Autodesk Inventor part; units mm, degrees
(part 3 of 3)
  line L1793 (-13.4182, -23.4177) -> (-13.3812, -23.2649)
  line L1794 (-13.3812, -23.2649) -> (-13.3062, -22.9928)
  line L1795 (-13.3062, -22.9928) -> (-13.2108, -22.6965)
  line L1796 (-13.2108, -22.6965) -> (-13.192, -22.6208)
  line L1797 (-13.192, -22.6208) -> (-13.1819, -22.5545)
  line L1798 (-13.1819, -22.5545) -> (-13.1803, -22.4978)
  line L1799 (-13.1803, -22.4978) -> (-13.1866, -22.4511)
  line L1800 (-13.1866, -22.4511) -> (-13.2004, -22.4146)
  line L1801 (-13.2004, -22.4146) -> (-13.2213, -22.3887)
  line L1802 (-13.2213, -22.3887) -> (-13.2509, -22.37)
  line L1803 (-13.2509, -22.37) -> (-13.4263, -22.2651)
  line L1804 (-13.4263, -22.2651) -> (-13.601, -22.1589)
  line L1805 (-13.601, -22.1589) -> (-13.6314, -22.1414)
  line L1806 (-13.6314, -22.1414) -> (-13.664, -22.135)
  line L1807 (-13.664, -22.135) -> (-13.7027, -22.1398)
  line L1808 (-13.7027, -22.1398) -> (-13.747, -22.1561)
  line L1809 (-13.747, -22.1561) -> (-13.7963, -22.184)
  line L1810 (-13.7963, -22.184) -> (-13.8503, -22.2238)
  line L1811 (-13.8503, -22.2238) -> (-13.9085, -22.2757)
  line L1812 (-13.9085, -22.2757) -> (-14.126, -22.4984)
  line L1813 (-14.126, -22.4984) -> (-14.3317, -22.6917)
  line L1814 (-14.3317, -22.6917) -> (-14.4495, -22.7958)
  line L1815 (-14.4495, -22.7958) -> (-14.5782, -22.9048)
  line L1816 (-14.5782, -22.9048) -> (-14.7187, -23.0187)
  line L1817 (-14.7187, -23.0187) -> (-14.8697, -23.1361)
  line L1818 (-14.8697, -23.1361) -> (-15.0319, -23.2568)
  line L1819 (-15.0319, -23.2568) -> (-15.2066, -23.3812)
  line L1820 (-15.2066, -23.3812) -> (-15.393, -23.5081)
  line L1821 (-15.393, -23.5081) -> (-15.5922, -23.6378)
  line L1822 (-15.5922, -23.6378) -> (-15.7628, -23.7441)
  arc A47 (-16.4074, -23.3034) -> (-15.7628, -23.7441) centre (0, 0) ccw
  line L1823 (-16.4074, -23.3034) -> (-16.3702, -23.1058)
  line L1824 (-16.3702, -23.1058) -> (-16.3217, -22.8731)
  line L1825 (-16.3217, -22.8731) -> (-16.271, -22.6533)
  line L1826 (-16.271, -22.6533) -> (-16.2185, -22.4455)
  line L1827 (-16.2185, -22.4455) -> (-16.1649, -22.2505)
  line L1828 (-16.1649, -22.2505) -> (-16.1103, -22.0672)
  line L1829 (-16.1103, -22.0672) -> (-16.055, -21.8949)
  line L1830 (-16.055, -21.8949) -> (-16.0002, -21.7355)
  line L1831 (-16.0002, -21.7355) -> (-15.946, -21.5879)
  line L1832 (-15.946, -21.5879) -> (-15.8404, -21.3261)
  line L1833 (-15.8404, -21.3261) -> (-15.7118, -21.0426)
  line L1834 (-15.7118, -21.0426) -> (-15.6846, -20.9696)
  line L1835 (-15.6846, -20.9696) -> (-15.667, -20.9048)
  line L1836 (-15.667, -20.9048) -> (-15.6589, -20.8487)
  line L1837 (-15.6589, -20.8487) -> (-15.6598, -20.8016)
  line L1838 (-15.6598, -20.8016) -> (-15.6694, -20.7638)
  line L1839 (-15.6694, -20.7638) -> (-15.6872, -20.7357)
  line L1840 (-15.6872, -20.7357) -> (-15.7145, -20.7137)
  line L1841 (-15.7145, -20.7137) -> (-15.8768, -20.5895)
  line L1842 (-15.8768, -20.5895) -> (-16.0383, -20.4641)
  line L1843 (-16.0383, -20.4641) -> (-16.0665, -20.4432)
  line L1844 (-16.0665, -20.4432) -> (-16.0982, -20.4331)
  line L1845 (-16.0982, -20.4331) -> (-16.1372, -20.4335)
  line L1846 (-16.1372, -20.4335) -> (-16.183, -20.4446)
  line L1847 (-16.183, -20.4446) -> (-16.2352, -20.4667)
  line L1848 (-16.2352, -20.4667) -> (-16.2934, -20.5001)
  line L1849 (-16.2934, -20.5001) -> (-16.3571, -20.5451)
  line L1850 (-16.3571, -20.5451) -> (-16.5986, -20.7415)
  line L1851 (-16.5986, -20.7415) -> (-16.8249, -20.9101)
  line L1852 (-16.8249, -20.9101) -> (-16.9539, -21.0001)
  line L1853 (-16.9539, -21.0001) -> (-17.0941, -21.0937)
  line L1854 (-17.0941, -21.0937) -> (-17.2467, -21.1909)
  line L1855 (-17.2467, -21.1909) -> (-17.4101, -21.2903)
  line L1856 (-17.4101, -21.2903) -> (-17.585, -21.3917)
  line L1857 (-17.585, -21.3917) -> (-17.7727, -21.4954)
  line L1858 (-17.7727, -21.4954) -> (-17.9724, -21.6002)
  line L1859 (-17.9724, -21.6002) -> (-18.1851, -21.7063)
  line L1860 (-18.1851, -21.7063) -> (-18.3667, -21.7925)
  arc A48 (-18.9569, -21.2812) -> (-18.3667, -21.7925) centre (0, 0) ccw
  line L1861 (-18.9569, -21.2812) -> (-18.8974, -21.0891)
  line L1862 (-18.8974, -21.0891) -> (-18.8226, -20.8635)
  line L1863 (-18.8226, -20.8635) -> (-18.7472, -20.6509)
  line L1864 (-18.7472, -20.6509) -> (-18.6714, -20.4504)
  line L1865 (-18.6714, -20.4504) -> (-18.5959, -20.2628)
  line L1866 (-18.5959, -20.2628) -> (-18.5207, -20.0869)
  line L1867 (-18.5207, -20.0869) -> (-18.4462, -19.9221)
  line L1868 (-18.4462, -19.9221) -> (-18.3736, -19.7699)
  line L1869 (-18.3736, -19.7699) -> (-18.3029, -19.6295)
  line L1870 (-18.3029, -19.6295) -> (-18.1682, -19.3814)
  line L1871 (-18.1682, -19.3814) -> (-18.0081, -19.1145)
  line L1872 (-18.0081, -19.1145) -> (-17.9727, -19.045)
  line L1873 (-17.9727, -19.045) -> (-17.9479, -18.9827)
  line L1874 (-17.9479, -18.9827) -> (-17.9334, -18.9278)
  line L1875 (-17.9334, -18.9278) -> (-17.929, -18.8809)
  line L1876 (-17.929, -18.8809) -> (-17.9342, -18.8423)
  line L1877 (-17.9342, -18.8423) -> (-17.9487, -18.8123)
  line L1878 (-17.9487, -18.8123) -> (-17.9733, -18.7874)
  line L1879 (-17.9733, -18.7874) -> (-18.1204, -18.6454)
  line L1880 (-18.1204, -18.6454) -> (-18.2665, -18.5024)
  line L1881 (-18.2665, -18.5024) -> (-18.2921, -18.4786)
  line L1882 (-18.2921, -18.4786) -> (-18.3224, -18.4649)
  line L1883 (-18.3224, -18.4649) -> (-18.3612, -18.4608)
  line L1884 (-18.3612, -18.4608) -> (-18.408, -18.4666)
  line L1885 (-18.408, -18.4666) -> (-18.4624, -18.4826)
  line L1886 (-18.4624, -18.4826) -> (-18.524, -18.5092)
  line L1887 (-18.524, -18.5092) -> (-18.5924, -18.5466)
  line L1888 (-18.5924, -18.5466) -> (-18.8547, -18.7142)
  line L1889 (-18.8547, -18.7142) -> (-19.0988, -18.856)
  line L1890 (-19.0988, -18.856) -> (-19.2372, -18.9306)
  line L1891 (-19.2372, -18.9306) -> (-19.3872, -19.0076)
  line L1892 (-19.3872, -19.0076) -> (-19.5499, -19.0868)
  line L1893 (-19.5499, -19.0868) -> (-19.7236, -19.1669)
  line L1894 (-19.7236, -19.1669) -> (-19.9089, -19.2477)
  line L1895 (-19.9089, -19.2477) -> (-20.1072, -19.3293)
  line L1896 (-20.1072, -19.3293) -> (-20.3175, -19.4107)
  line L1897 (-20.3175, -19.4107) -> (-20.5409, -19.4919)
  line L1898 (-20.5409, -19.4919) -> (-20.7311, -19.5568)
  arc A49 (-21.2592, -18.9815) -> (-20.7311, -19.5568) centre (0, 0) ccw
  line L1899 (-21.2592, -18.9815) -> (-21.1782, -18.7975)
  line L1900 (-21.1782, -18.7975) -> (-21.0782, -18.5819)
  line L1901 (-21.0782, -18.5819) -> (-20.9791, -18.3793)
  line L1902 (-20.9791, -18.3793) -> (-20.8808, -18.1887)
  line L1903 (-20.8808, -18.1887) -> (-20.7844, -18.011)
  line L1904 (-20.7844, -18.011) -> (-20.6898, -17.8448)
  line L1905 (-20.6898, -17.8448) -> (-20.5969, -17.6895)
  line L1906 (-20.5969, -17.6895) -> (-20.5074, -17.5466)
  line L1907 (-20.5074, -17.5466) -> (-20.4212, -17.4152)
  line L1908 (-20.4212, -17.4152) -> (-20.2591, -17.1841)
  line L1909 (-20.2591, -17.1841) -> (-20.0696, -16.9371)
  line L1910 (-20.0696, -16.9371) -> (-20.0265, -16.8721)
  line L1911 (-20.0265, -16.8721) -> (-19.9948, -16.813)
  line L1912 (-19.9948, -16.813) -> (-19.9741, -16.7602)
  line L1913 (-19.9741, -16.7602) -> (-19.9644, -16.7141)
  line L1914 (-19.9644, -16.7141) -> (-19.9651, -16.6751)
  line L1915 (-19.9651, -16.6751) -> (-19.9761, -16.6437)
  line L1916 (-19.9761, -16.6437) -> (-19.9977, -16.6161)
  line L1917 (-19.9977, -16.6161) -> (-20.1277, -16.4583)
  line L1918 (-20.1277, -16.4583) -> (-20.2565, -16.2996)
  line L1919 (-20.2565, -16.2996) -> (-20.2793, -16.273)
  line L1920 (-20.2793, -16.273) -> (-20.3079, -16.2559)
  line L1921 (-20.3079, -16.2559) -> (-20.3459, -16.2475)
  line L1922 (-20.3459, -16.2475) -> (-20.393, -16.2479)
  line L1923 (-20.393, -16.2479) -> (-20.4489, -16.2576)
  line L1924 (-20.4489, -16.2576) -> (-20.5132, -16.277)
  line L1925 (-20.5132, -16.277) -> (-20.5854, -16.3063)
  line L1926 (-20.5854, -16.3063) -> (-20.8651, -16.443)
  line L1927 (-20.8651, -16.443) -> (-21.1238, -16.5559)
  line L1928 (-21.1238, -16.5559) -> (-21.2697, -16.6144)
  line L1929 (-21.2697, -16.6144) -> (-21.4275, -16.6737)
  line L1930 (-21.4275, -16.6737) -> (-21.5982, -16.7339)
  line L1931 (-21.5982, -16.7339) -> (-21.7799, -16.7937)
  line L1932 (-21.7799, -16.7937) -> (-21.9732, -16.8528)
  line L1933 (-21.9732, -16.8528) -> (-22.1795, -16.9113)
  line L1934 (-22.1795, -16.9113) -> (-22.3977, -16.9682)
  line L1935 (-22.3977, -16.9682) -> (-22.6289, -17.0233)
  line L1936 (-22.6289, -17.0233) -> (-22.8253, -17.0662)
  arc A50 (-23.2843, -16.4344) -> (-22.8253, -17.0662) centre (0, 0) ccw
  line L1937 (-23.2843, -16.4344) -> (-23.1829, -16.2609)
  line L1938 (-23.1829, -16.2609) -> (-23.059, -16.058)
  line L1939 (-23.059, -16.058) -> (-22.9374, -15.8681)
  line L1940 (-22.9374, -15.8681) -> (-22.8181, -15.6899)
  line L1941 (-22.8181, -15.6899) -> (-22.7021, -15.5243)
  line L1942 (-22.7021, -15.5243) -> (-22.5891, -15.37)
  line L1943 (-22.5891, -15.37) -> (-22.4791, -15.2263)
  line L1944 (-22.4791, -15.2263) -> (-22.3739, -15.0946)
  line L1945 (-22.3739, -15.0946) -> (-22.2732, -14.9738)
  line L1946 (-22.2732, -14.9738) -> (-22.0858, -14.7627)
  line L1947 (-22.0858, -14.7627) -> (-21.8695, -14.5389)
  line L1948 (-21.8695, -14.5389) -> (-21.8192, -14.4793)
  line L1949 (-21.8192, -14.4793) -> (-21.781, -14.4242)
  line L1950 (-21.781, -14.4242) -> (-21.7545, -14.3741)
  line L1951 (-21.7545, -14.3741) -> (-21.7395, -14.3294)
  line L1952 (-21.7395, -14.3294) -> (-21.7358, -14.2906)
  line L1953 (-21.7358, -14.2906) -> (-21.7431, -14.2581)
  line L1954 (-21.7431, -14.2581) -> (-21.7615, -14.2282)
  line L1955 (-21.7615, -14.2282) -> (-21.8726, -14.0567)
  line L1956 (-21.8726, -14.0567) -> (-21.9825, -13.8843)
  line L1957 (-21.9825, -13.8843) -> (-22.002, -13.8552)
  line L1958 (-22.002, -13.8552) -> (-22.0285, -13.8351)
  line L1959 (-22.0285, -13.8351) -> (-22.0654, -13.8223)
  line L1960 (-22.0654, -13.8223) -> (-22.1122, -13.8174)
  line L1961 (-22.1122, -13.8174) -> (-22.1689, -13.8206)
  line L1962 (-22.1689, -13.8206) -> (-22.2349, -13.8325)
  line L1963 (-22.2349, -13.8325) -> (-22.31, -13.8535)
  line L1964 (-22.31, -13.8535) -> (-22.6034, -13.9573)
  line L1965 (-22.6034, -13.9573) -> (-22.8733, -14.0401)
  line L1966 (-22.8733, -14.0401) -> (-23.025, -14.0815)
  line L1967 (-23.025, -14.0815) -> (-23.1885, -14.1225)
  line L1968 (-23.1885, -14.1225) -> (-23.3649, -14.1628)
  line L1969 (-23.3649, -14.1628) -> (-23.5522, -14.2015)
  line L1970 (-23.5522, -14.2015) -> (-23.751, -14.2382)
  line L1971 (-23.751, -14.2382) -> (-23.9626, -14.2728)
  line L1972 (-23.9626, -14.2728) -> (-24.1859, -14.3044)
  line L1973 (-24.1859, -14.3044) -> (-24.4219, -14.3329)
  line L1974 (-24.4219, -14.3329) -> (-24.6219, -14.3531)
  arc A51 (-25.0059, -13.6731) -> (-24.6219, -14.3531) centre (0, 0) ccw
  line L1975 (-25.0059, -13.6731) -> (-24.8854, -13.5122)
  line L1976 (-24.8854, -13.5122) -> (-24.7391, -13.3248)
  line L1977 (-24.7391, -13.3248) -> (-24.5967, -13.15)
  line L1978 (-24.5967, -13.15) -> (-24.4579, -12.9866)
  line L1979 (-24.4579, -12.9866) -> (-24.3237, -12.8353)
  line L1980 (-24.3237, -12.8353) -> (-24.1939, -12.6949)
  line L1981 (-24.1939, -12.6949) -> (-24.0683, -12.5647)
  line L1982 (-24.0683, -12.5647) -> (-23.9487, -12.4458)
  line L1983 (-23.9487, -12.4458) -> (-23.8349, -12.3373)
  line L1984 (-23.8349, -12.3373) -> (-23.6247, -12.1489)
  line L1985 (-23.6247, -12.1489) -> (-23.3842, -11.9512)
  line L1986 (-23.3842, -11.9512) -> (-23.3275, -11.8977)
  line L1987 (-23.3275, -11.8977) -> (-23.2832, -11.8473)
  line L1988 (-23.2832, -11.8473) -> (-23.2512, -11.8005)
  line L1989 (-23.2512, -11.8005) -> (-23.2312, -11.7578)
  line L1990 (-23.2312, -11.7578) -> (-23.2231, -11.7197)
  line L1991 (-23.2231, -11.7197) -> (-23.2267, -11.6866)
  line L1992 (-23.2267, -11.6866) -> (-23.2415, -11.6549)
  line L1993 (-23.2415, -11.6549) -> (-23.3324, -11.4717)
  line L1994 (-23.3324, -11.4717) -> (-23.4219, -11.288)
  line L1995 (-23.4219, -11.288) -> (-23.438, -11.2569)
  line L1996 (-23.438, -11.2569) -> (-23.462, -11.2338)
  line L1997 (-23.462, -11.2338) -> (-23.4972, -11.2169)
  line L1998 (-23.4972, -11.2169) -> (-23.5432, -11.2067)
  line L1999 (-23.5432, -11.2067) -> (-23.5998, -11.2035)
  line L2000 (-23.5998, -11.2035) -> (-23.6668, -11.2078)
  line L2001 (-23.6668, -11.2078) -> (-23.7437, -11.22)
  line L2002 (-23.7437, -11.22) -> (-24.0471, -11.2898)
  line L2003 (-24.0471, -11.2898) -> (-24.3247, -11.3412)
  line L2004 (-24.3247, -11.3412) -> (-24.4801, -11.3651)
  line L2005 (-24.4801, -11.3651) -> (-24.6472, -11.3871)
  line L2006 (-24.6472, -11.3871) -> (-24.827, -11.4071)
  line L2007 (-24.827, -11.4071) -> (-25.0175, -11.4242)
  line L2008 (-25.0175, -11.4242) -> (-25.2192, -11.438)
  line L2009 (-25.2192, -11.438) -> (-25.4334, -11.4482)
  line L2010 (-25.4334, -11.4482) -> (-25.6588, -11.4542)
  line L2011 (-25.6588, -11.4542) -> (-25.8966, -11.4556)
  line L2012 (-25.8966, -11.4556) -> (-26.0976, -11.4528)
  arc A52 (-26.4016, -10.7335) -> (-26.0976, -11.4528) centre (0, 0) ccw
  line L2013 (-26.4016, -10.7335) -> (-26.2634, -10.5874)
  line L2014 (-26.2634, -10.5874) -> (-26.0968, -10.4179)
  line L2015 (-26.0968, -10.4179) -> (-25.9354, -10.2604)
  line L2016 (-25.9354, -10.2604) -> (-25.7788, -10.1139)
  line L2017 (-25.7788, -10.1139) -> (-25.6283, -9.979)
  line L2018 (-25.6283, -9.979) -> (-25.4833, -9.8542)
  line L2019 (-25.4833, -9.8542) -> (-25.3437, -9.7392)
  line L2020 (-25.3437, -9.7392) -> (-25.2113, -9.6347)
  line L2021 (-25.2113, -9.6347) -> (-25.0859, -9.5399)
  line L2022 (-25.0859, -9.5399) -> (-24.8556, -9.3767)
  line L2023 (-24.8556, -9.3767) -> (-24.5942, -9.2077)
  line L2024 (-24.5942, -9.2077) -> (-24.5317, -9.161)
  line L2025 (-24.5317, -9.161) -> (-24.482, -9.116)
  line L2026 (-24.482, -9.116) -> (-24.4448, -9.0732)
  line L2027 (-24.4448, -9.0732) -> (-24.4201, -9.033)
  line L2028 (-24.4201, -9.033) -> (-24.4077, -8.9961)
  line L2029 (-24.4077, -8.9961) -> (-24.4075, -8.9628)
  line L2030 (-24.4075, -8.9628) -> (-24.4186, -8.9296)
  line L2031 (-24.4186, -8.9296) -> (-24.488, -8.7373)
  line L2032 (-24.488, -8.7373) -> (-24.556, -8.5445)
  line L2033 (-24.556, -8.5445) -> (-24.5684, -8.5118)
  line L2034 (-24.5684, -8.5118) -> (-24.5896, -8.4861)
  line L2035 (-24.5896, -8.4861) -> (-24.6226, -8.4654)
  line L2036 (-24.6226, -8.4654) -> (-24.6672, -8.4499)
  line L2037 (-24.6672, -8.4499) -> (-24.7231, -8.4403)
  line L2038 (-24.7231, -8.4403) -> (-24.7901, -8.4369)
  line L2039 (-24.7901, -8.4369) -> (-24.868, -8.4403)
  line L2040 (-24.868, -8.4403) -> (-25.1773, -8.475)
  line L2041 (-25.1773, -8.475) -> (-25.4589, -8.4945)
  line L2042 (-25.4589, -8.4945) -> (-25.616, -8.5005)
  line L2043 (-25.616, -8.5005) -> (-25.7846, -8.5033)
  line L2044 (-25.7846, -8.5033) -> (-25.9655, -8.5027)
  line L2045 (-25.9655, -8.5027) -> (-26.1567, -8.4979)
  line L2046 (-26.1567, -8.4979) -> (-26.3587, -8.4887)
  line L2047 (-26.3587, -8.4887) -> (-26.5726, -8.4744)
  line L2048 (-26.5726, -8.4744) -> (-26.7973, -8.4547)
  line L2049 (-26.7973, -8.4547) -> (-27.0336, -8.4289)
  line L2050 (-27.0336, -8.4289) -> (-27.233, -8.4033)
  arc A53 (-27.453, -7.654) -> (-27.233, -8.4033) centre (0, 0) ccw
  line L2051 (-27.453, -7.654) -> (-27.2991, -7.5246)
  line L2052 (-27.2991, -7.5246) -> (-27.1142, -7.3752)
  line L2053 (-27.1142, -7.3752) -> (-26.9359, -7.2371)
  line L2054 (-26.9359, -7.2371) -> (-26.7637, -7.1095)
  line L2055 (-26.7637, -7.1095) -> (-26.5988, -6.9925)
  line L2056 (-26.5988, -6.9925) -> (-26.4405, -6.8851)
  line L2057 (-26.4405, -6.8851) -> (-26.2886, -6.7867)
  line L2058 (-26.2886, -6.7867) -> (-26.1452, -6.698)
  line L2059 (-26.1452, -6.698) -> (-26.0099, -6.6181)
  line L2060 (-26.0099, -6.6181) -> (-25.7624, -6.4823)
  line L2061 (-25.7624, -6.4823) -> (-25.4834, -6.3442)
  line L2062 (-25.4834, -6.3442) -> (-25.4161, -6.3049)
  line L2063 (-25.4161, -6.3049) -> (-25.3615, -6.2659)
  line L2064 (-25.3615, -6.2659) -> (-25.3197, -6.2276)
  line L2065 (-25.3197, -6.2276) -> (-25.2906, -6.1905)
  line L2066 (-25.2906, -6.1905) -> (-25.2741, -6.1552)
  line L2067 (-25.2741, -6.1552) -> (-25.2701, -6.1221)
  line L2068 (-25.2701, -6.1221) -> (-25.2773, -6.0879)
  line L2069 (-25.2773, -6.0879) -> (-25.3243, -5.8889)
  line L2070 (-25.3243, -5.8889) -> (-25.3699, -5.6896)
  line L2071 (-25.3699, -5.6896) -> (-25.3785, -5.6557)
  line L2072 (-25.3785, -5.6557) -> (-25.3967, -5.6278)
  line L2073 (-25.3967, -5.6278) -> (-25.4271, -5.6034)
  line L2074 (-25.4271, -5.6034) -> (-25.4696, -5.583)
  line L2075 (-25.4696, -5.583) -> (-25.524, -5.5671)
  line L2076 (-25.524, -5.5671) -> (-25.5902, -5.5561)
  line L2077 (-25.5902, -5.5561) -> (-25.668, -5.5506)
  line L2078 (-25.668, -5.5506) -> (-25.9793, -5.5498)
  line L2079 (-25.9793, -5.5498) -> (-26.2613, -5.537)
  line L2080 (-26.2613, -5.537) -> (-26.418, -5.525)
  line L2081 (-26.418, -5.525) -> (-26.5858, -5.5087)
  line L2082 (-26.5858, -5.5087) -> (-26.7655, -5.4874)
  line L2083 (-26.7655, -5.4874) -> (-26.9549, -5.4609)
  line L2084 (-26.9549, -5.4609) -> (-27.1545, -5.4287)
  line L2085 (-27.1545, -5.4287) -> (-27.3654, -5.3901)
  line L2086 (-27.3654, -5.3901) -> (-27.5864, -5.3449)
  line L2087 (-27.5864, -5.3449) -> (-27.8182, -5.2924)
  line L2088 (-27.8182, -5.2924) -> (-28.0134, -5.2442)
  arc A54 (-28.1465, -4.4747) -> (-28.0134, -5.2442) centre (0, 0) ccw
  line L2089 (-28.1465, -4.4747) -> (-27.9789, -4.3637)
  line L2090 (0, 3.4641) -> (3, 1.7321)
  line L2091 (3, 1.7321) -> (3, -1.7321)
  line L2092 (3, -1.7321) -> (0, -3.4641)
  line L2093 (0, -3.4641) -> (-3, -1.7321)
  line L2094 (-3, -1.7321) -> (-3, 1.7321)
  line L2095 (-3, 1.7321) -> (0, 3.4641)
  arc A55 (-3.3489, 7.8125) -> (-3.3489, 20.7313) centre (-27.5, 14.2719) ccw
  arc A56 (3.3489, 20.7313) -> (3.3489, 7.8125) centre (27.5, 14.2719) ccw
  arc A57 (-8.465, -0.7708) -> (-20.7515, 3.2213) centre (-22.0713, -21.7438) ccw
  arc A58 (-18.6817, 9.5913) -> (-6.3953, 5.5992) centre (-5.0754, 30.5643) ccw
  arc A59 (-1.8828, -8.2889) -> (-9.4762, -18.7404) centre (13.8592, -27.7103) ccw
  arc A60 (-14.8948, -14.8035) -> (-7.3014, -4.352) centre (-30.6368, 4.6179) ccw
  arc A61 (7.3014, -4.352) -> (14.8948, -14.8035) centre (30.6368, 4.6179) ccw
  arc A62 (9.4762, -18.7404) -> (1.8828, -8.2889) centre (-13.8592, -27.7103) ccw
  arc A63 (6.3953, 5.5992) -> (18.6817, 9.5913) centre (5.0754, 30.5643) ccw
  arc A64 (20.7515, 3.2213) -> (8.465, -0.7708) centre (22.0713, -21.7438) ccw
  arc A65 (-3.3489, 7.8125) -> (-6.3953, 5.5992) centre (0, 0) ccw
  arc A66 (-8.465, -0.7708) -> (-7.3014, -4.352) centre (0, 0) ccw
  arc A67 (-3.3489, 20.7313) -> (-18.6817, 9.5913) centre (0, 0) ccw
  arc A68 (18.6817, 9.5913) -> (3.3489, 20.7313) centre (0, 0) ccw
  arc A69 (-1.8828, -8.2889) -> (1.8828, -8.2889) centre (0, 0) ccw
  arc A70 (7.3014, -4.352) -> (8.465, -0.7708) centre (0, 0) ccw
  arc A71 (6.3953, 5.5992) -> (3.3489, 7.8125) centre (0, 0) ccw
  arc A72 (14.8948, -14.8035) -> (20.7515, 3.2213) centre (0, 0) ccw
  arc A73 (-20.7515, 3.2213) -> (-14.8948, -14.8035) centre (0, 0) ccw
  arc A74 (-9.4762, -18.7404) -> (9.4762, -18.7404) centre (0, 0) ccw
  point P0 (3, 0)
  dimension "d3" = 6
  dimension "d10" = 25
  dimension "d11" = 25
  dimension "d12" = 5
  dimension "d15" = 360
  dimension "d17" = 8.5
  dimension "d18" = 21
  constraints: 4192 end point, 40 point on circle, 20 centre point, 3 horizontal alignment, 3 vertical alignment, 2 coincident, 1 midpoint, 220 other
  measures "d3" distance of L2091.end L2093.end
  measures "d10" radius of A55
  measures "d11" radius of A56
  measures "d17" radius of A71
  measures "d18" radius of A68
extrude "Extrusión3" add sketch "Boceto4" along normal blind 6
